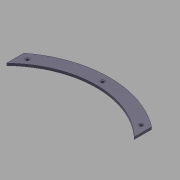
# Autodesk Inventor part: BaseCover
Saved by Autodesk Inventor 2017 (Build 210142000, 142)
## iProperties
Created: 2017-05-08
Part Number: BaseCover
Material: ABS Plastic
Document SubType Name: Modeling
Designer: zallen
Density: 1.06 g/cm^3
Appearance: Default Plastic
Mass: 72.8492 g
Surface Area: 267.673 cm^2
Volume: 68.7257 cm^3
Author: zallen
Autodesk Inventor part; units mm, degrees
ref_plane "YZ Plane" through (0, 0, 0) normal (1, 0, 0) x (0, 1, 0)
ref_plane "XZ Plane" through (0, 0, 0) normal (0, 1, 0) x (-1, 0, 0)
ref_plane "XY Plane" through (0, 0, 0) normal (0, 0, 1) x (1, 0, 0)
sketch "Sketch14" plane through (0, 0, 0) normal (0, 0, 1) x (1, 0, 0)
  line L0 (-139.2442, -85) -> (-139.2442, -47.3019)
  line L1 (0, 0) -> (0, -356.2475) construction
  line L2 (0, 0) -> (-146.5249, 0) construction
  circle A0 centre (0, -228.6) radius 228.6 construction
  arc A1 (0, 0) -> (-139.2442, -47.3019) centre (0.2992, -229.4806) ccw
  arc A2 (0, -28.6152) -> (-139.2442, -85) centre (0.2992, -229.4806) ccw
  line L3 (139.2442, -85) -> (139.2442, -47.3019)
  arc A3 (139.2442, -47.3019) -> (0, 0) centre (-0.2992, -229.4806) ccw
  arc A4 (139.2442, -85) -> (0, -28.6152) centre (-0.2992, -229.4806) ccw
  circle A5 centre (0, -15) radius 7.5
  circle A6 centre (-124, -55) radius 7.5
  circle A7 centre (124, -55) radius 7.5
  circle A8 centre (-124, -55) radius 2.5
  circle A9 centre (0, -15) radius 2.5
  circle A10 centre (124, -55) radius 2.5
  dimension "d152" = 139.2442
  dimension "d153" = 85
  dimension "d155" = 457.2
  dimension "d156" = 200.8656
  dimension "d159" = 15
  dimension "d160" = 15
  dimension "d161" = 15
  dimension "d162" = 55
  dimension "d163" = 124
  dimension "d164" = 5
  dimension "d165" = 5
  dimension "d166" = 5
  constraints: 11 centre point, 11 point on circle, 10 end point, 5 symmetric about line, 4 coincident, 3 point on line, 2 vertical, 1 concentric, 1 horizontal, 3 other
  measures "d152" distance between parallel lines of L1 L0
  measures "d153" vertical distance of L1.start L0.start
  measures "d155" diameter of A0
  measures "d156" radius of A2
  measures "d159" diameter of A5
  measures "d160" distance of A1.start A5.centre
  measures "d161" diameter of A6
  measures "d162" vertical distance of A1.start A6.centre
  measures "d163" horizontal distance of A1.start A6.centre
  measures "d164" diameter of A8
  measures "d165" diameter of A9
  measures "d166" diameter of A10
extrude "Extrusion14" add sketch "Sketch14" along normal blind 5 contours L0 A1 A3 L3 A4 A2 | A5 | A6 | A7
fillet "Fillet2" radius 2 3 edges at (-126.5, -55, 5) (-2.5, -15, 5) (121.5, -55, 5)
body "Solid4"
